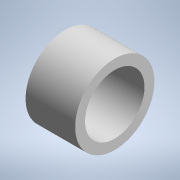
# Autodesk Inventor part: PACK-WSJJ8-6-5
Saved by Autodesk Inventor 2020 (Build 240168000, 168)
## iProperties
Part Number: PACK-WSJJ8-6-5
Material: 一般
Catalog Web Link: www.cadenas.de
Description: PACK-WSJJ,PACK-WSJM-Resin Washer Bulk Packages - Standard
Vendor: MISUMI
Document SubType Name: Modeling
Designer: partserver
Manufacturer: MISUMI
Mass: 0.109956 g
Surface Area: 2.63894 cm^2
Volume: 0.109956 cm^3
Density: 1 g/cm^3
Appearance: PSOLRGB-255-255-255
Category: PARTsolutions
Company: MISUMI
PSOL_IDENT_0: {$CADENAS_DATA\23d-libs\misumi\metric\26_washers_collars\pack_wsjj.prj},191 {VTYP=3D},{NB=PACK-WSJJ8
PSOL_IDENT_1: -6-5},{LINA=PACK-WSJJ8-6-5},{NN=PACK-WSJJ,PACK-WSJM},{DATE=07.06.2021 03:25:42},{GEOMDATE=02.03.2017
PSOL_IDENT_2: 08:58:00},{VERSION=},{LINEID=40},{WBVAR=MAT,V,T},{WBNUMERIC=V,T}  {NB=PACK-WSJJ8-6-5},{LINA=PACK-WS
PSOL_IDENT_3: JJ8-6-5},{KT=DUMMY},{PN=PACK-WSJJ8-6-5},{TYPE=PACK-WSJJ},{D=8},{MAT=1},{MATALG='1', 'Polyacetal', '2'
PSOL_IDENT_4: , 'MC Nylon Standard Grade' },{COLOR=White},{COLOR2=1.00,1.00,1.00,0.00},{V=6},{VALG=[3:6/1]},{T=5},
PSOL_IDENT_5: {TALG=[2:3/1],[5]}
NB: PACK-WSJJ8-6-5
NN: PACK-WSJJ,PACK-WSJM
NT: Resin Washer Bulk Packages - Standard
NBSYN: $PN.
LINA: PACK-WSJJ8-6-5
CATALOG: Misumi
PN: PACK-WSJJ8-6-5
D: 8
MAT: Polyacetal
COLOR: White
V: 6
T: 5
SUPPLIER: MISUMI
ARTICLENO: PACK-WSJJ8-6-5
BOMINFO: PACK-WSJJ8-6-5
CREATOR: CADENAS GmbH
Title: PACK-WSJJ8-6-5
Author: Cadenas PARTsolutions
Comments: Resin Washer Bulk Packages - Standard
Autodesk Inventor part; units mm, degrees
ref_plane "YZ Plane" through (0, 0, 0) normal (1, 0, 0) x (0, 1, 0)
ref_plane "XZ Plane" through (0, 0, 0) normal (0, 1, 0) x (-1, 0, 0)
ref_plane "XY Plane" through (0, 0, 0) normal (0, 0, 1) x (1, 0, 0)
sketch "_____1" plane through (0, 0, 0) normal (0, 0, 1) x (1, 0, 0)
  line L0 (2.5, 0) -> (-2.5, 0)
  line L1 (-2.5, 4) -> (-2.5, 3)
  line L2 (-2.5, 3) -> (2.5, 3)
  line L3 (2.5, 3) -> (2.5, 4)
  line L4 (2.5, 4) -> (-2.5, 4)
  constraints: 10 end point
revolve "Revolution1" add sketch "_____1" angle 360 about axis through (2.5, 0, 0) along (1, 0, 0)
body "Solid1"
